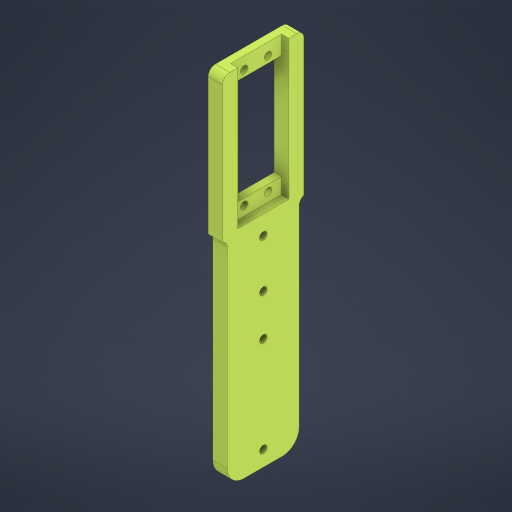
# Autodesk Inventor part: antebrazo_1
Saved by Autodesk Inventor 2023.1 (Build 271208000, 208)
## iProperties
Created: 2022-10-22
Part Number: antebrazo_1
Material: Generic
Document SubType Name: Modeling
Designer: amtat
Density: 1 g/cm^3
Appearance: Default
Author: amtat
Autodesk Inventor part; units mm, degrees
ref_plane "YZ Plane" through (0, 0, 0) normal (1, 0, 0) x (0, 1, 0)
ref_plane "XZ Plane" through (0, 0, 0) normal (0, 1, 0) x (-1, 0, 0)
ref_plane "XY Plane" through (0, 0, 0) normal (0, 0, 1) x (1, 0, 0)
sketch "Sketch1" plane through (0, 0, 0) normal (1, 0, 0) x (0, 1, 0)
  line L0 (0, 0) -> (0, -30)
  line L1 (0, -30) -> (150, -30)
  line L2 (150, -30) -> (150, 0)
  line L3 (150, 0) -> (0, 0)
  dimension "d0" = 30
  dimension "d1" = 150
  constraints: 8 end point, 1 horizontal, 1 parallel, 1 perpendicular, 1 vertical
  measures "d0" distance of L0.start L0.end
  measures "d1" distance of L0.end L1.end
extrude "Extrusion1" add sketch "Sketch1" along normal blind 3
sketch "Sketch2" plane through (3, 0, 0) normal (1, 0, 0) x (0, 0, -1)
  line L0 (30, 0) -> (30, 150) projected
  line L1 (30, 150) -> (0, 150) projected
  line L2 (0, 150) -> (0, 0) projected
  line L3 (0, 0) -> (30, 0) projected
  line L4 (30, 150) -> (0, 150) projected
  line L5 (0, 150) -> (0, 145)
  line L6 (0, 150) -> (0, 0) projected
  line L7 (0, 145) -> (30, 145)
  line L8 (30, 0) -> (30, 150) projected
  line L9 (0, 145) -> (15, 145)
  line L10 (15, 145) -> (20, 145)
  line L11 (15, 145) -> (10, 145)
  circle A0 centre (10, 145) radius 1.5
  circle A1 centre (20, 145) radius 1.5
  circle A2 centre (20, 95.8) radius 1.5
  circle A3 centre (10, 95.8) radius 1.5
  line L12 (20, 95.8) -> (20, 97.3)
  line L13 (20, 143.5) -> (20, 145)
  line L14 (10, 95.8) -> (11.5, 95.8)
  line L15 (18.5, 95.8) -> (20, 95.8)
  line L16 (10, 145) -> (10, 143.5)
  line L17 (10, 97.3) -> (10, 95.8)
  line L18 (15, 145) -> (15, 120.4)
  line L19 (15, 120.4) -> (15, 140.9)
  line L20 (15, 140.9) -> (25.15, 140.9)
  line L21 (25.15, 140.9) -> (25.15, 99.9)
  line L22 (25.15, 99.9) -> (4.85, 99.9)
  line L23 (4.85, 99.9) -> (4.85, 140.9)
  line L24 (4.85, 140.9) -> (15, 140.9)
  dimension "d8" = 3
  dimension "d9" = 3
  dimension "d4" = 5
  dimension "d5" = 15
  dimension "d6" = 5
  dimension "d7" = 5
  dimension "d10" = 49.2
  dimension "d11" = 3
  dimension "d12" = 3
  dimension "d15" = 24.6
  dimension "d16" = 20.5
  dimension "d17" = 10.15
  dimension "d18" = 41
  dimension "d19" = 20.3
  constraints: 36 end point, 8 perpendicular, 5 point on line, 4 coincident, 4 point on circle, 2 centre point, 2 parallel, 2 vertical, 2 vertical alignment, 1 horizontal, 1 midpoint, 4 other
  measures "d4" distance of L1.end L5.end
  measures "d5" distance of L5.end L9.end
  measures "d6" distance of L9.end L10.end
  measures "d7" distance of L9.end L11.end
  measures "d10" distance of L16.start L14.start
  measures "d11" diameter of A2
  measures "d12" diameter of A3
  measures "d15" distance of L9.end L18.end
  measures "d16" distance of L18.end L19.end
  measures "d17" distance of L19.end L20.end
  measures "d18" distance of L20.end L21.end
  measures "d19" distance of L21.end L22.end
extrude "Extrusion2" cut sketch "Sketch2" against normal through all contours A1 L13 L7 | L7 A1 | L13 A1 L7 | A0 L7 | L7 L16 A0 | L7 A0 L16 | A2 L15 L12 | L12 L15 A2 | L14 L17 A3 | A3 L17 L14 | L20 L21 L22 L23 L24
sketch "Sketch3" plane through (3, 0, 0) normal (1, 0, 0) x (0, 0, -1)
  circle A0 centre (20, 145) radius 1.5 projected
  circle A1 centre (10, 95.8) radius 1.5 projected
  circle A2 centre (10, 145) radius 1.5 projected
  circle A3 centre (20, 95.8) radius 1.5 projected
  line L0 (25.15, 140.9) -> (25.15, 99.9) projected
  line L1 (25.15, 99.9) -> (4.85, 99.9) projected
  line L2 (4.85, 99.9) -> (4.85, 140.9) projected
  line L3 (4.85, 140.9) -> (25.15, 140.9) projected
  line L4 (30, 0) -> (30, 150) projected
  line L5 (30, 150) -> (0, 150) projected
  line L6 (0, 150) -> (0, 0) projected
  line L7 (0, 0) -> (30, 0) projected
  line L8 (20, 95.8) -> (15, 95.8)
  line L9 (15, 95.8) -> (15, 85.8)
  circle A4 centre (15, 85.8) radius 1.5
  line L10 (15, 85.8) -> (15, 65.8)
  circle A5 centre (15, 65.8) radius 1.5
  line L11 (20, 95.8) -> (20, 91.8)
  line L12 (20, 91.8) -> (25.15, 91.8)
  line L13 (25.15, 91.8) -> (25.15, 99.9)
  line L14 (20, 91.8) -> (4.85, 91.8)
  line L15 (25.15, 99.9) -> (4.85, 99.9) projected
  line L16 (4.85, 91.8) -> (4.85, 99.9)
  line L17 (25.15, 99.9) -> (25.15, 150)
  line L18 (30, 150) -> (0, 150) projected
  line L19 (4.85, 99.9) -> (4.85, 150)
  dimension "d22" = 5
  dimension "d23" = 10
  dimension "d24" = 3
  dimension "d34" = 20
  dimension "d35" = 3
  dimension "d41" = 4
  constraints: 20 end point, 6 perpendicular, 2 centre point, 2 coincident, 2 horizontal, 2 point on line, 2 vertical
  measures "d22" distance of L8.start L8.end
  measures "d23" distance of L8.end L9.end
  measures "d24" diameter of A4
  measures "d34" distance of L10.start L10.end
  measures "d35" diameter of A5
  measures "d41" distance of L8.start L11.end
extrude "Extrusion7" add sketch "Sketch3" along normal blind 3 contours L12 L13 L0 L17 L5 L4 L7 L6 L19 L2 L16 L14 | A4 L10 L9 | L9 L10 A4 | A5
sketch "Sketch5" plane through (0, 0, 0) normal (-1, 0, 0) x (0, 0, 1)
  circle A0 centre (-20, 145) radius 1.5 projected
  circle A1 centre (-10, 95.8) radius 1.5 projected
  circle A2 centre (-10, 145) radius 1.5 projected
  circle A3 centre (-20, 95.8) radius 1.5 projected
  line L0 (-25.15, 99.9) -> (-25.15, 140.9) projected
  line L1 (-25.15, 140.9) -> (-4.85, 140.9) projected
  line L2 (-4.85, 140.9) -> (-4.85, 99.9) projected
  line L3 (-4.85, 99.9) -> (-25.15, 99.9) projected
  line L4 (-30, 0) -> (-30, 150) projected
  line L5 (0, 0) -> (-30, 0) projected
  line L6 (0, 150) -> (0, 0) projected
  line L7 (-30, 150) -> (0, 150) projected
  line L8 (0, 146) -> (0, 0) projected
  line L9 (0, 0) -> (-15, 0)
  line L10 (0, 0) -> (-30, 0) projected
  line L11 (-15, 0) -> (-15, 6.5)
  circle A4 centre (-15, 6.5) radius 1.5
  line L12 (-15, 6.5) -> (-15, 46.5)
  circle A5 centre (-15, 46.5) radius 1.5
  dimension "d45" = 15
  dimension "d46" = 6.5
  dimension "d47" = 3
  dimension "d48" = 40
  dimension "d49" = 3
  constraints: 6 end point, 2 centre point, 2 coincident, 1 midpoint, 1 perpendicular, 1 point on line
  measures "d45" distance of L8.end L9.end
  measures "d46" distance of L9.end L11.end
  measures "d47" diameter of A4
  measures "d48" distance of L12.start L12.end
  measures "d49" diameter of A5
extrude "Extrusion8" cut sketch "Sketch5" against normal blind 10 contours A4 L12 L11 | L11 L12 A4 | A5
sketch "Sketch6" plane through (6, 0, 0) normal (1, 0, 0) x (0, 0, -1)
  circle A0 centre (15, 6.5) radius 1.5 projected
  circle A1 centre (15, 46.5) radius 1.5 projected
  line L0 (30, 150) -> (25.15, 150) projected
  line L1 (25.15, 150) -> (25.15, 91.8) projected
  line L2 (25.15, 91.8) -> (4.85, 91.8) projected
  line L3 (4.85, 91.8) -> (4.85, 150) projected
  line L4 (4.85, 150) -> (0, 150) projected
  line L5 (0, 150) -> (0, 0) projected
  line L6 (0, 0) -> (30, 0) projected
  line L7 (30, 0) -> (30, 150) projected
  line L8 (25.15, 91.8) -> (25.15, 99.9) projected
  line L9 (25.15, 99.9) -> (4.85, 99.9) projected
  line L10 (4.85, 99.9) -> (4.85, 91.8) projected
  line L11 (4.85, 91.8) -> (25.15, 91.8) projected
  circle A2 centre (10, 95.8) radius 1.5 projected
  circle A3 centre (20, 95.8) radius 1.5 projected
  circle A4 centre (20, 95.8) radius 1.5 projected
  line L12 (20, 95.8) -> (15, 95.8)
  line L13 (15, 95.8) -> (15, 91.8)
  line L14 (25.15, 91.8) -> (4.85, 91.8) projected
  line L15 (15, 91.8) -> (15, 88.8)
  line L16 (15, 88.8) -> (15, 83.8)
  line L17 (15, 83.8) -> (15, 63.8)
  circle A5 centre (15, 63.8) radius 1.5
  circle A6 centre (15, 83.8) radius 1.5
  dimension "d52" = 5
  dimension "d53" = 3
  dimension "d54" = 5
  dimension "d55" = 20
  dimension "d56" = 3
  dimension "d57" = 3
  constraints: 10 end point, 3 point on line, 2 centre point, 2 coincident, 1 horizontal, 1 midpoint
  measures "d52" distance of L12.start L12.end
  measures "d53" distance of L13.end L15.end
  measures "d54" distance of L15.end L16.end
  measures "d55" distance of L16.end L17.end
  measures "d56" diameter of A5
  measures "d57" diameter of A6
extrude "Extrusion9" cut sketch "Sketch6" against normal blind 10 contours A6 L17 L16 | L16 L17 A6 | A5
sketch "Sketch8" plane through (6, 0, 0) normal (1, 0, 0) x (0, 0, -1)
  circle A0 centre (15, 63.8) radius 1.5 projected
  circle A1 centre (15, 83.8) radius 1.5 projected
  circle A2 centre (15, 6.5) radius 1.5 projected
  circle A3 centre (15, 46.5) radius 1.5 projected
  line L0 (30, 150) -> (25.15, 150) projected
  line L1 (25.15, 150) -> (25.15, 91.8) projected
  line L2 (25.15, 91.8) -> (4.85, 91.8) projected
  line L3 (4.85, 91.8) -> (4.85, 150) projected
  line L4 (4.85, 150) -> (0, 150) projected
  line L5 (0, 150) -> (0, 0) projected
  line L6 (0, 0) -> (30, 0) projected
  line L7 (30, 0) -> (30, 150) projected
  line L8 (4.85, 91.8) -> (25.15, 91.8) projected
  line L9 (25.15, 91.8) -> (25.65, 91.8)
  line L10 (25.65, 91.8) -> (25.65, 150)
  line L11 (26, 150) -> (4, 150) projected
  line L12 (4.85, 91.8) -> (4.35, 91.8)
  line L13 (4.35, 91.8) -> (4.35, 150)
  line L14 (4.85, 150) -> (4, 150) projected
  dimension "d60" = 0.5
  dimension "d61" = 0.5
  constraints: 8 end point, 3 point on line, 2 perpendicular, 1 horizontal
  measures "d60" distance of L1.end L9.end
  measures "d61" distance of L2.end L12.end
extrude "Extrusion10" cut sketch "Sketch8" against normal blind 3 contours L10 L9 L1 L0 | L3 L12 L13 L4
sketch "Sketch9" plane through (3, 0, 0) normal (1, 0, 0) x (0, 0, -1)
  line L0 (4.35, 91.8) -> (25.65, 91.8) projected
  line L1 (25.65, 150) -> (25.65, 91.8) projected
  line L2 (25.65, 150) -> (4.35, 150) projected
  line L3 (4.35, 91.8) -> (4.35, 150) projected
  circle A0 centre (20, 145) radius 1.5 projected
  circle A1 centre (10, 145) radius 1.5 projected
  line L4 (4.85, 140.9) -> (4.85, 99.9) projected
  line L5 (4.85, 140.9) -> (25.15, 140.9) projected
  line L6 (25.15, 99.9) -> (25.15, 140.9) projected
  line L7 (25.15, 99.9) -> (4.85, 99.9) projected
  circle A2 centre (10, 95.8) radius 1.5 projected
  circle A3 centre (20, 95.8) radius 1.5 projected
  circle A4 centre (15, 46.5) radius 1.5 projected
  circle A5 centre (15, 6.5) radius 1.5 projected
  circle A6 centre (15, 83.8) radius 1.5 projected
  circle A7 centre (15, 63.8) radius 1.5 projected
  line L8 (25.65, 91.8) -> (4.35, 91.8) projected
  line L9 (4.35, 91.8) -> (4.35, 150) projected
  line L10 (4.35, 150) -> (0, 150) projected
  line L11 (0, 150) -> (0, 0) projected
  line L12 (0, 0) -> (30, 0) projected
  line L13 (30, 0) -> (30, 150) projected
  line L14 (30, 150) -> (25.65, 150) projected
  line L15 (25.65, 150) -> (25.65, 91.8) projected
  line L16 (4.85, 140.9) -> (25.15, 140.9) projected
  line L17 (4.85, 140.9) -> (4.35, 140.9)
  line L18 (25.15, 99.9) -> (25.15, 140.9) projected
  line L19 (25.15, 140.9) -> (25.65, 140.9)
  line L20 (25.65, 150) -> (25.65, 91.8) projected
  line L21 (25.15, 99.9) -> (4.85, 99.9) projected
  line L22 (25.15, 99.9) -> (25.65, 99.9)
  line L23 (4.85, 99.9) -> (4.35, 99.9)
  constraints: 8 end point, 6 point on line, 1 collinear, 1 perpendicular
extrude "Extrusion11" cut sketch "Sketch9" against normal blind 3 contours L3 L17 L4 L23 | L22 L6 L19 L1
sketch "Sketch10" plane through (3, 0, 0) normal (1, 0, 0) x (0, 0, -1)
  line L0 (4.35, 140.9) -> (25.65, 140.9) projected
  line L1 (25.65, 150) -> (25.65, 140.9) projected
  line L2 (25.65, 150) -> (4.35, 150) projected
  line L3 (4.35, 140.9) -> (4.35, 150) projected
  circle A0 centre (10, 145) radius 1.5 projected
  circle A1 centre (20, 145) radius 1.5 projected
  line L4 (25.65, 99.9) -> (4.35, 99.9) projected
  line L5 (4.35, 91.8) -> (4.35, 99.9) projected
  line L6 (4.35, 91.8) -> (25.65, 91.8) projected
  line L7 (25.65, 99.9) -> (25.65, 91.8) projected
  circle A2 centre (10, 95.8) radius 1.5 projected
  circle A3 centre (20, 95.8) radius 1.5 projected
  line L8 (4.35, 140.9) -> (4.35, 141.9)
  line L9 (4.35, 91.8) -> (4.35, 150) projected
  line L10 (25.65, 150) -> (25.65, 91.8) projected
  line L11 (25.65, 140.9) -> (25.65, 141.9)
  line L12 (4.35, 99.9) -> (4.35, 99.4)
  line L13 (4.35, 99.4) -> (25.65, 99.4)
  line L14 (25.65, 99.9) -> (25.65, 99.4)
  line L15 (4.35, 140.9) -> (4.35, 141.4)
  line L16 (4.35, 141.4) -> (25.65, 141.4)
  line L17 (25.65, 141.4) -> (25.65, 140.9)
  point P0 (0, 0)
  dimension "d67" = 0.5
  dimension "d68" = 0.5
  constraints: 16 end point, 5 point on line, 2 collinear, 2 perpendicular, 1 midpoint
  measures "d67" distance of L4.end L12.end
  measures "d68" distance of L0.start L15.end
extrude "Extrusion12" cut sketch "Sketch10" against normal blind 3 contours L3 L16 L1 L0 | L4 L7 L13 L5
sketch "Sketch11" plane through (3, 0, 0) normal (1, 0, 0) x (0, 0, -1)
  circle A0 centre (20, 145) radius 1.5 projected
  circle A1 centre (10, 145) radius 1.5 projected
  line L0 (4.35, 141.4) -> (25.65, 141.4) projected
  line L1 (25.65, 150) -> (25.65, 141.4) projected
  line L2 (25.65, 150) -> (4.35, 150) projected
  line L3 (4.35, 141.4) -> (4.35, 150) projected
  line L4 (25.65, 99.4) -> (4.35, 99.4) projected
  line L5 (4.35, 91.8) -> (4.35, 99.4) projected
  line L6 (4.35, 91.8) -> (25.65, 91.8) projected
  line L7 (25.65, 99.4) -> (25.65, 91.8) projected
  circle A2 centre (10, 95.8) radius 1.5 projected
  circle A3 centre (20, 95.8) radius 1.5 projected
  circle A4 centre (10, 95.8) radius 1.5 projected
  line L8 (10, 97.3) -> (10, 98.5)
  line L9 (10, 98.5) -> (25.65, 98.5)
  line L10 (25.65, 150) -> (25.65, 91.8) projected
  line L11 (10, 98.5) -> (4.35, 98.5)
  line L12 (4.35, 91.8) -> (4.35, 150) projected
  circle A5 centre (10, 145) radius 1.5 projected
  line L13 (10, 143.5) -> (10, 142.3)
  line L14 (10, 142.3) -> (25.65, 142.3)
  line L15 (10, 142.3) -> (4.35, 142.3)
  point P0 (0, 0)
  point P1 (4.35, 142.3)
  point P2 (4.35, 98.5)
  dimension "d71" = 1.2
  dimension "d72" = 1.2
  constraints: 12 end point, 6 point on line, 4 perpendicular, 2 vertical alignment, 2 other
  measures "d71" distance of L8.start L8.end
  measures "d72" distance of L13.start L13.end
extrude "Extrusion13" cut sketch "Sketch11" against normal blind 3 contours L3 L15 L14 L1 L0 | L4 L7 L9 L11 L5
sketch "Sketch12" plane through (0, 0, -30) normal (0, 0, -1) x (-1, 0, 0)
  line L0 (0, 0) -> (0, 150) projected
  line L1 (0, 150) -> (-6, 150) projected
  line L2 (-6, 0) -> (-6, 150) projected
  line L3 (0, 0) -> (-6, 0) projected
  line L4 (-6, 150) -> (-6, 90)
  line L5 (-6, 0) -> (-6, 150) projected
  line L6 (-6, 90) -> (0, 90)
  line L7 (0, 0) -> (0, 150) projected
  dimension "d75" = 60
  constraints: 4 end point, 2 point on line, 1 horizontal
  measures "d75" distance of L1.end L4.end
extrude "Extrusion14" add sketch "Sketch12" along normal blind 2 contours L6 L2 L1 L0
sketch "Sketch13" plane through (0, 0, 0) normal (0, 0, 1) x (1, 0, 0)
  line L0 (0, 150) -> (0, 0) projected
  line L1 (0, 0) -> (6, 0) projected
  line L2 (6, 150) -> (6, 0) projected
  line L3 (0, 150) -> (6, 150) projected
  line L4 (6, 150) -> (6, 90) projected
  line L5 (6, 150) -> (6, 90)
  line L6 (6, 90) -> (0, 90)
  dimension "d78" = 60
  constraints: 4 end point, 1 collinear, 1 perpendicular, 1 point on line
  measures "d78" distance of L2.start L4.end
extrude "Extrusion15" add sketch "Sketch13" along normal blind 2 contours L3 L2 L6 L0
fillet "Fillet3" radius 3 2 edges at (3, 150, 2) (3, 150, -32)
fillet "Fillet4" radius 3 2 edges at (3, 90, 0) (3, 90, -30)
fillet "Fillet5" radius 7 2 edges at (3, 0, -30) (3, 0, 0)
body "Solid1"
